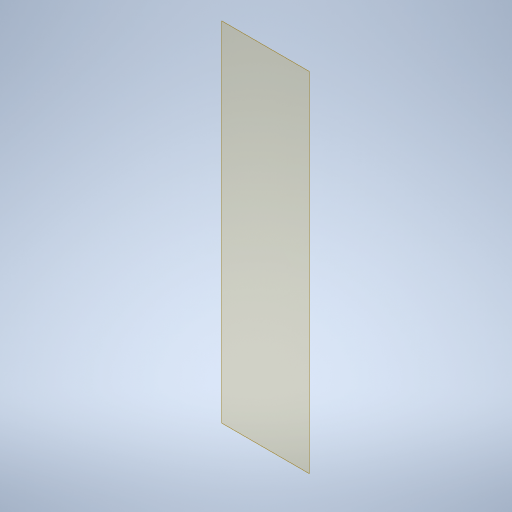
# Autodesk Inventor part: top-tensioner
Saved by Autodesk Inventor 2024 (Build 280153000, 153)
## iProperties
Created: 2024-04-14
Part Number: top-tensioner
Material: Generic
Document SubType Name: Modeling
Designer: MaartenGeorgesBuelen
Density: 1 g/cm^3
Appearance: Default
Author: MaartenGeorgesBuelen
## iProperties of the stored document top-tensioner_3DPrint.ipt
Created: 2024-04-14
Part Number: top-tensioner_3DPrint
Material: Generic
Document SubType Name: Modeling
Designer: MaartenGeorgesBuelen
Density: 1 g/cm^3
Appearance: Default
Author: MaartenGeorgesBuelen
Autodesk Inventor part; units mm, degrees
note: some values were not read from the file. Chosen so that the rebuilt part matches the saved one: edges of "Fillet3".
ref_plane "YZ Plane" through (0, 0, 0) normal (1, 0, 0) x (0, 1, 0)
ref_plane "XZ Plane" through (0, 0, 0) normal (0, 1, 0) x (-1, 0, 0)
ref_plane "XY Plane" through (0, 0, 0) normal (0, 0, 1) x (1, 0, 0)
ref_plane "Work Plane1" through (0, 0, 0) normal (0, 0, 1) x (1, 0, 0)
sketch "Sketch1" plane through (0, 0, 0) normal (0, 0, 1) x (1, 0, 0)
  circle A0 centre (-15.435, 47.2375) radius 1.95 projected
  circle A1 centre (-15.435, 57.2375) radius 1.95 projected
  circle A2 centre (15.435, 47.2375) radius 1.95 projected
  circle A3 centre (15.435, 57.2375) radius 1.95 projected
  circle A4 centre (0, -62.5) radius 13.5 projected
  circle A5 centre (0, -43.5) radius 2 projected
  circle A6 centre (-13.435, -49.065) radius 2 projected
  circle A7 centre (13.435, -49.065) radius 2 projected
  circle A8 centre (-13.435, -75.935) radius 2 projected
  arc A9 (-14.8492, -77.3492) -> (0, -83.5) centre (0, -62.5) ccw projected
  circle A10 centre (0, -81.5) radius 2 projected
  arc A11 (0, -83.5) -> (14.8492, -77.3492) centre (0, -62.5) ccw projected
  circle A12 centre (13.435, -75.935) radius 2 projected
  arc A13 (14.8492, -77.3492) -> (21, -62.5) centre (0, -62.5) ccw projected
  circle A14 centre (19, -62.5) radius 2 projected
  line L0 (21, 62.5) -> (21, -62.5) projected
  arc A15 (21, 62.5) -> (-21, 62.5) centre (0, 62.5) ccw projected
  line L1 (-21, -62.5) -> (-21, 62.5) projected
  circle A16 centre (-19, -62.5) radius 2 projected
  arc A17 (-21, -62.5) -> (-14.8492, -77.3492) centre (0, -62.5) ccw projected
  circle A18 centre (-15.5, -1.9727) radius 2.1 projected
  circle A19 centre (15.5, -1.9727) radius 2.1 projected
  circle A20 centre (-15.5, 29.0273) radius 2.1 projected
  circle A21 centre (15.5, 29.0273) radius 2.1 projected
  circle A22 centre (0, 13.5273) radius 13 projected
  line L2 (11.435, 61.2375) -> (19.435, 61.2375)
  line L3 (19.435, 61.2375) -> (19.435, 43.2375)
  line L4 (19.435, 43.2375) -> (11.435, 43.2375)
  line L5 (11.435, 43.2375) -> (11.435, 61.2375)
  circle A23 centre (15.435, 57.2375) radius 2.35
  circle A24 centre (15.435, 47.2375) radius 2.35
  line L6 (11.435, 43.2375) -> (17.0919, 37.5807)
  line L7 (11.435, 43.2375) -> (19.435, 43.2375) construction
  line L8 (19.435, 43.2375) -> (25.0919, 37.5807)
  line L9 (17.0919, 37.5807) -> (26.0919, 37.5807)
  line L10 (26.0919, 37.5807) -> (26.0919, 26.5807)
  line L11 (26.0919, 26.5807) -> (17.0919, 26.5807)
  line L12 (17.0919, 26.5807) -> (17.0919, 37.5807)
  point P0 (0, 0)
  dimension "d0" = 4
  dimension "d1" = 4
  dimension "d2" = 4
  dimension "d3" = 4
  dimension "d4" = 0.4
  dimension "d5" = 0.4
  dimension "d6" = 8
  dimension "d7" = 45
  dimension "d8" = 11
  dimension "d19" = 9
  constraints: 22 end point, 5 parallel, 3 horizontal, 2 centre point, 2 equal length, 2 horizontal alignment, 2 perpendicular, 1 vertical alignment, 2 other
  measures "d0" distance from line of L3 A2.centre
  measures "d1" distance from line of L5 A2.centre
  measures "d2" distance from line of L2 A3.centre
  measures "d3" distance from line of L4 A2.centre
  measures "d4" radial gap between concentric circles of A3 A23
  measures "d5" radial gap between concentric circles of A2 A24
  measures "d6" distance of L4.end L6.end
  measures "d7" angle of L6 L7
  measures "d8" distance of L9.end L10.end
  measures "d19" distance of L10.end L11.end
extrude "Extrusion1" add sketch "Sketch1" along normal blind 4 contours L11 L12 A21 L9 L0 | L0 L9 L10 L11 | L8 L9 L0 | L0 L9 L6 L4 L8 | L4 L5 L2 L3 | L12 A21 picked at (17.2417, 29.1915)
sketch "Sketch2" plane through (0, 0, 4) normal (0, 0, 1) x (1, 0, 0)
  line L0 (19.435, 61.2375) -> (11.435, 61.2375) projected
  line L1 (11.435, 61.2375) -> (11.435, 43.2375) projected
  line L2 (11.435, 43.2375) -> (17.0919, 37.5807) projected
  line L3 (17.0919, 37.5807) -> (17.0919, 26.5807) projected
  line L4 (17.0919, 26.5807) -> (26.0919, 26.5807) projected
  line L5 (26.0919, 26.5807) -> (26.0919, 37.5807) projected
  line L6 (25.0919, 37.5807) -> (19.435, 43.2375) projected
  line L7 (19.435, 43.2375) -> (19.435, 61.2375) projected
  circle A0 centre (15.435, 47.2375) radius 2.35 projected
  circle A1 centre (15.435, 57.2375) radius 2.35 projected
  line L8 (17.0919, 26.5807) -> (25.0919, 26.5807)
  line L9 (25.0919, 26.5807) -> (25.0919, 37.5807)
  line L10 (25.0919, 37.5807) -> (17.0919, 37.5807)
  line L11 (17.0919, 37.5807) -> (17.0919, 26.5807)
  line L12 (26.0919, 37.5807) -> (25.0919, 37.5807) projected
  point P0 (0, 0)
  point P1 (25.0919, 26.5807)
  constraints: 8 end point, 2 parallel, 1 horizontal, 1 perpendicular
extrude "Extrusion2" add sketch "Sketch2" along normal blind 9 contours L12 L5 L4 L9 | L9 L4 L3 L10
sketch "Sketch3" plane through (26.0919, 26.5807, 0) normal (1, 0, 0) x (0, 0, -1)
  line L0 (0, 0) -> (0, 11) projected
  line L1 (-13, 0) -> (-13, 11) projected
  line L2 (0, 0) -> (-13, 0) projected
  circle A0 centre (-8, 5.5) radius 2.85
  line L3 (0, 11) -> (-13, 11) projected
  point P0 (0, -26.5807)
  dimension "d13" = 8
  dimension "d14" = 5.5
  dimension "d15" = 5.7
  constraints: 1 centre point
  measures "d13" distance from line of L0 A0.centre
  measures "d14" distance from line of L2 A0.centre
  measures "d15" diameter of A0
fillet "Fillet1" radius 2 4 edges at (11.435, 43.2375, 2) (11.435, 61.2375, 2) (19.435, 61.2375, 2) (19.435, 43.2375, 2)
extrude "Extrusion3" cut sketch "Sketch3" against normal through all contours A0
fillet "Fillet2" radius 2 2 edges at (21.5919, 37.5807, 13) (21.5919, 26.5807, 13)
fillet "Fillet3" radius 1 10 edges at (17.0919, 27.1665, 12.4142) (17.0919, 32.0807, 13) (17.0919, 36.9949, 12.4142) (17.0919, 37.5807, 7.5) (17.0919, 26.5807, 5.5) (26.0919, 27.1665, 12.4142) (26.0919, 32.0807, 13) (26.0919, 36.9949, 12.4142) (26.0919, 37.5807, 5.5) (26.0919, 26.5807, 5.5)
body "Solid1"
